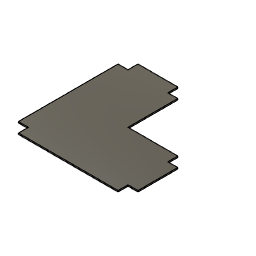
_ShelfL.3a8be7bf-2398-4533-8ec0-87d4e1979ddc (Autodesk Fusion 360 design; units mm, degrees)
Autodesk Fusion 360 part; units mm, degrees
sketch "Sketch1" plane through (0, 0, 0) normal (0, 0, 1) x (1, 0, 0)
  line L0 (0, 0) -> (0, 609.6)
  line L1 (0, 609.6) -> (304.8, 609.6)
  line L2 (304.8, 609.6) -> (304.8, 304.8)
  line L3 (304.8, 304.8) -> (609.6, 304.8)
  line L4 (609.6, 304.8) -> (609.6, 0)
  line L5 (609.6, 0) -> (0, 0)
  line L6 (609.6, 0) -> (558.8, 0)
  line L7 (558.8, 0) -> (558.8, 50.8)
  line L8 (558.8, 50.8) -> (609.6, 50.8)
  line L9 (609.6, 50.8) -> (609.6, 0)
  line L10 (609.6, 304.8) -> (558.8, 304.8)
  line L11 (558.8, 304.8) -> (558.8, 254)
  line L12 (558.8, 254) -> (609.6, 254)
  line L13 (609.6, 254) -> (609.6, 304.8)
  line L14 (0, 0) -> (50.8, 0)
  line L15 (50.8, 0) -> (50.8, 50.8)
  line L16 (50.8, 50.8) -> (0, 50.8)
  line L17 (0, 50.8) -> (0, 0)
  line L18 (0, 609.6) -> (50.8, 609.6)
  line L19 (50.8, 609.6) -> (50.8, 558.8)
  line L20 (50.8, 558.8) -> (0, 558.8)
  line L21 (0, 558.8) -> (0, 609.6)
  line L22 (304.8, 609.6) -> (254, 609.6)
  line L23 (254, 609.6) -> (254, 558.8)
  line L24 (254, 558.8) -> (304.8, 558.8)
  line L25 (304.8, 558.8) -> (304.8, 609.6)
  dimension "d1" = 304.8
  dimension "d2" = 609.6
  dimension "d3" = 304.8
  dimension "d4" = 609.6
  dimension "d7" = 50.8
  dimension "d8" = 50.8
  dimension "d9" = 50.8
  dimension "d10" = 50.8
  dimension "d11" = 50.8
  dimension "d12" = 50.8
  constraint coincident L0.start L5.end
  constraint vertical L0
  constraint perpendicular L0 L1
  constraint perpendicular L1 L2
  constraint perpendicular L2 L3
  constraint perpendicular L1 L4
  constraint perpendicular L0 L5
  constraint horizontal L6
  constraint vertical L7
  constraint horizontal L8
  constraint vertical L9
  constraint horizontal L10
  constraint vertical L11
  constraint horizontal L12
  constraint vertical L13
  constraint horizontal L14
  constraint vertical L15
  constraint horizontal L16
  constraint vertical L17
  constraint horizontal L18
  constraint vertical L19
  constraint horizontal L20
  constraint vertical L21
  constraint horizontal L22
  constraint vertical L23
  constraint horizontal L24
  constraint vertical L25
  constraint collinear L7 L11
  constraint collinear L8 L16
  constraint collinear L20 L24
  constraint collinear L15 L19
  measures "d1" distance of L3.end L4.end
  measures "d2" distance of L0.start L0.end
  measures "d3" distance of L0.end L1.end
  measures "d4" distance of L0.start L4.end
  measures "d7" distance of L10.end L11.end
  measures "d8" distance of L4.end L8.end
  measures "d9" distance of L11.end L12.end
  measures "d10" distance of L0.start L14.end
  measures "d11" distance of L1.end L24.end
  measures "d12" distance of L1.end L22.end
extrude "Extrude1" add sketch "Sketch1" along normal blind 6.35 contours L0 L1 L2 L3 L4 L5 L7 L8 L11 L12 L15 L16 L19 L20 L23 L24
